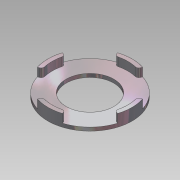
# Autodesk Inventor part: button_barrel
Saved by Autodesk Inventor 2019.3 (Build 233278000, 278)
## iProperties
Created: 2019-03-01
Part Number: button_barrel
Material: ABS Plastic
Document SubType Name: Modeling
Designer: WW
Density: 1.06 g/cm^3
Appearance: Smooth - White
Author: WW
Autodesk Inventor part; units mm, degrees
ref_plane "YZ Plane" through (0, 0, 0) normal (1, 0, 0) x (0, 1, 0)
ref_plane "XZ Plane" through (0, 0, 0) normal (0, 1, 0) x (-1, 0, 0)
ref_plane "XY Plane" through (0, 0, 0) normal (0, 0, 1) x (1, 0, 0)
sketch "Sketch1" plane through (0, 0, 0) normal (0, 1, 0) x (-1, 0, 0)
  circle A0 centre (0, 0) radius 30
  dimension "d0" = 60
  constraints: 1 centre point, 1 coincident
  measures "d0" diameter of A0
extrude "Extrusion1" add sketch "Sketch1" along normal blind 2.5
sketch "Sketch2" plane through (0, 2.5, 0) normal (0, 1, 0) x (1, 0, 0)
  circle A0 centre (0, 0) radius 30 projected
  circle A1 centre (0, 0) radius 27
  circle A2 centre (0, 0) radius 30 construction
  line L0 (-28.6529, -8.8889) -> (-25.7876, -8)
  line L1 (-25.7876, 8) -> (-28.6529, 8.8889)
  line L2 (-25.7876, -8) -> (-25.7876, 8) construction
  arc A3 (-28.6529, 8.8889) -> (-28.6529, -8.8889) centre (0, 0) ccw
  arc A4 (-25.7876, 8) -> (-25.7876, -8) centre (0, 0) ccw
  dimension "d3" = 3
  dimension "d4" = 16
  constraints: 8 point on circle, 6 end point, 3 centre point, 2 concentric, 2 point on line, 1 vertical
  measures "d3" radial gap between concentric circles of A0 A1
  measures "d4" distance of L0.end L1.start
extrude "Extrusion2" add sketch "Sketch2" along normal blind 6 contours L1 A1 L0 A0 picked at (-28.0966, 6.6307)
fillet "Fillet1" radius 2 2 edges at (-25.7876, 5.5, 8) (-25.7876, 5.5, -8)
pattern_circular "Circular Pattern1" count 4 over 360 about axis through (0, 0, 0) along (0, 1, 0) of "Fillet1", "Extrusion2"
sketch "Sketch3" plane through (0, 0, 0) normal (0, -1, 0) x (1, 0, 0)
  circle A0 centre (0, 0) radius 17
  dimension "d11" = 34
  constraints: 1 centre point, 1 coincident
  measures "d11" diameter of A0
extrude "Extrusion3" cut sketch "Sketch3" against normal through all
body "Solid1"
